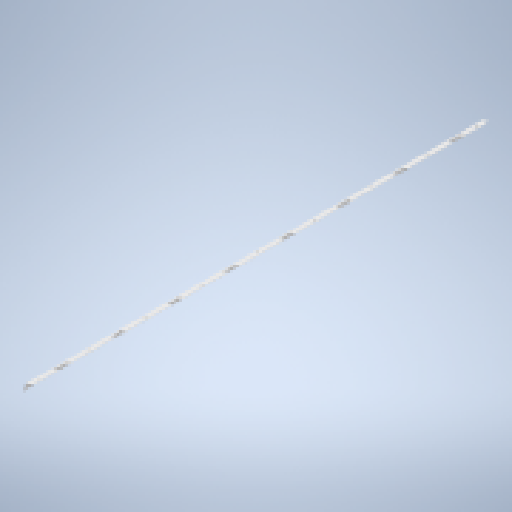
# Autodesk Inventor part: ДМФ 01 17 опора крышки
Saved by Autodesk Inventor 2024.2 (Build 282272000, 272)
## iProperties
Created: 2024-04-30
Part Number: ДМФ 01 17 опора крышки
Material: Generic
Document SubType Name: Sheet Metal
Designer: pokla
Density: 1 g/cm^3
Appearance: Default
Sheet Metal Rule: Default
Flat Pattern Width: 7.22619 cm
Flat Pattern Length: 202 cm
Flat Pattern Area: 1459.69 cm^2
Sheet Metal Width: 72,262 mm
Sheet Metal Length: 2020,000 mm
Sheet Metal Area: 145969,132 mm^2
Author: pokla
Autodesk Inventor part; units mm, degrees
ref_plane "YZ Plane" through (0, 0, 0) normal (1, 0, 0) x (0, 1, 0)
ref_plane "XZ Plane" through (0, 0, 0) normal (0, 1, 0) x (-1, 0, 0)
ref_plane "XY Plane" through (0, 0, 0) normal (0, 0, 1) x (1, 0, 0)
sketch "Sketch4" plane through (0, 0, 0) normal (0, 0, 1) x (1, 0, 0)
  line L0 (-192.87245, 192.87245) -> (0, 272.762834) construction
  line L1 (0, 272.762834) -> (192.87245, 192.87245) construction
  line L2 (192.87245, 192.87245) -> (272.762834, 0) construction
  line L3 (272.762834, 0) -> (192.87245, -192.87245) construction
  line L4 (192.87245, -192.87245) -> (0, -272.762834) construction
  line L5 (0, -272.762834) -> (-192.87245, -192.87245) construction
  line L6 (-192.87245, -192.87245) -> (-272.762834, 0) construction
  line L7 (-272.762834, 0) -> (-192.87245, 192.87245) construction
  line L8 (-272.128784, 1.530734) -> (-258.734864, 33.866517)
  line L9 (-272.128784, -1.530734) -> (-258.734864, -33.866517)
  arc A0 (-272.128784, 1.530734) -> (-272.128784, -1.530734) centre (-268.433266, 0) ccw
  point P0 (0, 0)
  point P1 (0, 0)
  point P2 (0, 0)
  dimension "d16" = 504
  dimension "d23" = 35
  dimension "d24" = 4
  measures "d16" distance between parallel lines of L7 L3
  measures "d23" distance of L8.start L8.end
  measures "d24" radius of A0
contour flange "Contour Flange1" sketch "Sketch4" thickness 2 bend radius 2 width 2020 along (0, 0, -1) mid plane no both sides no wall seen from (-265.431824, 17.698626, 0) lies toward (0.9238795, -0.3826834, 0) curves L8 A0 L9
bend "Bend2"
corner "Corner2"
sketch "Sketch6" plane through (-272.128784, 1.530734, 0) normal (-0.9238795, 0.3826834, 0) x (0.3826834, 0.9238795, 0)
  circle A0 centre (17.5, 40.75) radius 5.5
  line L0 (35, 0) -> (0, 0) projected
  circle A1 centre (17.5, 1979.25) radius 5.5
  line L1 (35, 2020) -> (0, 2020) projected
  point P0 (102.724963, 0)
  point P1 (17.5, 0)
  point P2 (17.5, 0)
  point P3 (17.5, 0)
  point P4 (17.5, 0)
  point P5 (17.5, 2020)
  point P6 (17.5, 2020)
  dimension "d36" = 11
  dimension "d37" = 40.75
  dimension "d40" = 40.75
  dimension "d41" = 11
  constraints: 6 midpoint, 2 centre point, 2 vertical alignment
  measures "d36" diameter of A0
  measures "d37" distance of point (17.5, 0) A0.centre
  measures "d40" distance of point (17.5, 2020) A1.centre
  measures "d41" diameter of A1
extrude "Extrusion1" cut sketch "Sketch6" against normal up to surface (2 mm away)
sketch "Sketch12" plane through (-272.128784, -1.530734, -2020) normal (-0.9238795, -0.3826834, 0) x (0, 0, 1)
  line L0 (860, -35) -> (910, -35) construction
  line L1 (910, -35) -> (910, -10) construction
  line L2 (910, -10) -> (860, -10) construction
  line L3 (860, -10) -> (860, -35) construction
  line L4 (2020, 0) -> (0, 0)
  line L5 (889.849742, -11.4) -> (894.699485, -19.8)
  line L6 (894.699485, -19.8) -> (889.849742, -28.2)
  line L7 (889.849742, -28.2) -> (880.150258, -28.2)
  line L8 (880.150258, -28.2) -> (875.300515, -19.8)
  line L9 (875.300515, -19.8) -> (880.150258, -11.4)
  line L10 (880.150258, -11.4) -> (889.849742, -11.4)
  point P0 (2020, -102.724963)
  point P1 (0, -35)
  point P2 (1010, 0)
  point P3 (885, -10)
  point P4 (885, -19.8)
  point P5 (885, -11.4)
  dimension "d75" = 50
  dimension "d76" = 25
  dimension "d77" = 125
  dimension "magic_d3" = 16.8
  dimension "magic_d2" = 19.8
  constraints: 20 end point, 3 midpoint, 2 parallel, 2 vertical alignment, 1 horizontal, 1 horizontal alignment, 1 perpendicular, 13 other
  measures "d75" distance of L0.start L0.end
  measures "d76" distance of L2.end L0.start
  measures "d77" horizontal distance of point (1010, 0) point (885, -10)
  measures "magic_d3" distance between parallel lines of L7 L10
  measures "magic_d2" distance from line of point (885, -19.8) L4
extrude "Extrusion6" cut sketch "Sketch12" against normal through all
mirror "Mirror1" about plane through (0, 0, 0) normal (0, 1, 0) of "Extrusion6"
pattern_linear "Rectangular Pattern4" count 8 spacing 250 along (0, 0, 1) of "Extrusion6", "Mirror1" first direction both ways yes
sketch "Sketch13" plane through (-272.128784, 1.530734, 0) normal (-0.9238795, 0.3826834, 0) x (0.3826834, 0.9238795, 0)
  circle A0 centre (16.3, 1010) radius 5.5
  line L0 (35, 0) -> (35, 2020) projected
  line L1 (35, 0) -> (0, 0) projected
  point P0 (102.724963, 0)
  point P1 (35, 1010)
  point P2 (35, 910)
  point P3 (35, 1110)
  point P4 (17.5, 0)
  dimension "d83" = 11
  dimension "magic_d1" = 18.7
  constraints: 2 midpoint, 1 centre point, 1 horizontal alignment
  measures "d83" diameter of A0
  measures "magic_d1" distance from line of A0.centre L0
extrude "Extrusion7" cut sketch "Sketch13" against normal through all
pattern_linear "Rectangular Pattern5" count 7 spacing 250 along (0, 0, 1) of "Extrusion7" first direction both ways yes
equation "\"d40\" = d37"
equation "\"d77\" = Барабан_Отступ_окна_от_середины"
equation "\"d16\" = Барабан_габарит_по_кассетам - Thickness"
equation "\"d24\" = BendRadius + Thickness"
equation "\"d41\" = d36"
equation "\"d75\" = Барабан_Ширина_окна"
equation "\"d25\" = Thickness"
equation "\"d26\" = BendReliefWidth"
equation "\"d27\" = BendReliefDepth"
equation "\"d28\" = MinimumRemnant"
equation "\"d29\" = TransitionRadius"
equation "\"d30\" = Барабан_длина_листа"
equation "\"d31\" = BendRadius"
equation "\"d33\" = CornerReliefSize"
equation "\"d34\" = GapSize"
equation "\"d35\" = JacobiRadiusSize"
equation "\"BendRadius\" = Thickness"
equation "\"BendReliefWidth\" = Thickness"
equation "\"BendReliefDepth\" = 0.5 * Thickness"
equation "\"CornerReliefSize\" = 4 * Thickness"
equation "\"MinimumRemnant\" = 2 * Thickness"
equation "\"TransitionRadius\" = BendRadius"
equation "\"JacobiRadiusSize\" = BendRadius"
equation "\"GapSize\" = Thickness"
equation "\"Барабан_габарит_по_кассетам\" = 506"
equation "\"Thickness\" = 2"
equation "\"Барабан_Ширина_окна\" = 50"
equation "\"Барабан_длина_листа\" = 2020"
equation "\"Барабан_Отступ_окна_от_середины\" = 125"
body "Solid2"
